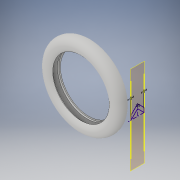
# Autodesk Inventor part: 複習二
Saved by Autodesk Inventor 2017 (Build 210142000, 142)
## iProperties
Part Number: 複習二
Material: 一般
Document SubType Name: Modeling
Designer: user
Density: 1 g/cm^3
Appearance: 預設
Author: user
Autodesk Inventor part; units mm, degrees
ref_plane "YZ Plane" through (0, 0, 0) normal (1, 0, 0) x (0, 1, 0)
ref_plane "XZ Plane" through (0, 0, 0) normal (0, 1, 0) x (-1, 0, 0)
ref_plane "XY Plane" through (0, 0, 0) normal (0, 0, 1) x (1, 0, 0)
sketch "草圖1" plane through (0, 0, 0) normal (0, 0, 1) x (1, 0, 0)
  arc A0 (-22.3939, -13.2104) -> (-22.3939, 13.2104) centre (0, 0) ccw
  arc A1 (-30.6227, -22.5) -> (-30.6227, 22.5) centre (0, 0) ccw
  line L0 (0, 0) -> (-32.9837, 0)
  line L1 (-22.3939, 22.5) -> (-30.6227, 22.5)
  line L2 (-22.3939, -22.5) -> (-30.6227, -22.5)
  line L3 (-30.6227, 22.5) -> (-30.6227, -28.3205)
  line L4 (-22.3939, 22.5) -> (-22.3939, 13.2104)
  line L5 (-22.3939, -13.2104) -> (-22.3939, -22.5)
  line L6 (0, -38) -> (-195, -38)
  line L7 (-195, 44.7459) -> (-195, -38)
  dimension "d0" = 52
  dimension "d1" = 76
  dimension "d2" = 45
  dimension "d12" = 195
  constraints: 16 end point, 5 point on circle, 3 horizontal, 3 vertical, 2 centre point, 2 coincident, 2 perpendicular, 1 symmetric about line, 1 tangent
  measures "d0" diameter of A0
  measures "d1" diameter of A1
  measures "d2" distance of L1.start L2.start
  measures "d12" distance of L6.start L6.end
revolve "迴轉2" add sketch "草圖1" angle 360 about axis through (-195, 44.7459, 0) along (0, -1, 0) contours A0 L4 L1 A1 L2 L5
ref_plane "工作平面2" through (110, 0, 0) normal (1, 0, 0) x (0, 1, 0)
sketch "草圖2" plane through (110, 0, 0) normal (1, 0, 0) x (0, 1, 0)
  line L0 (-38, 25) -> (0, 63)
  line L1 (0, 63) -> (38, 25)
  line L2 (38, 25) -> (38, 0)
  line L3 (38, 195) -> (38, -195) projected
  line L4 (38, 0) -> (0, 38)
  line L5 (0, 38) -> (-38, 0)
  line L6 (-38, 0) -> (-38, 25)
  line L7 (-38, 195) -> (-38, -195) projected
  line L8 (38, 0) -> (-54.583, 0)
  line L9 (0, 0) -> (0, 56.6709)
  dimension "d18" = 0
  dimension "d19" = 0
  dimension "d23" = 25
  constraints: 16 end point, 3 equal length, 2 collinear, 2 perpendicular, 2 point on line, 1 horizontal, 1 vertical
  measures "d18" distance between parallel lines of L7 L6
  measures "d19" distance between parallel lines of L3 L2
  measures "d23" distance of L0.end L4.end
